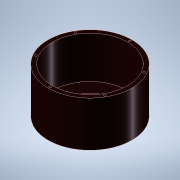
# Autodesk Inventor part: Top
Saved by Autodesk Inventor 2021 (Build 250183000, 183)
## iProperties
Created: 2022-09-01
Part Number: Top
Material: Ogólny
Document SubType Name: Modeling
Designer: MicnedSQ
Density: 1 g/cm^3
Appearance: Kasztanowa
Author: MicnedSQ
## iProperties of the stored document _Drukowanie 3D.ipt
Created: 2022-09-01
Part Number: _Drukowanie 3D
Material: Ogólny
Document SubType Name: Modeling
Designer: MicnedSQ
Density: 1 g/cm^3
Appearance: Domyślna
Author: MicnedSQ
Autodesk Inventor part; units mm, degrees
ref_plane "YZ Plane" through (0, 0, 0) normal (1, 0, 0) x (0, 1, 0)
ref_plane "XZ Plane" through (0, 0, 0) normal (0, 1, 0) x (-1, 0, 0)
ref_plane "XY Plane" through (0, 0, 0) normal (0, 0, 1) x (1, 0, 0)
sketch "Szkic1" plane through (0, 0, 0) normal (0, 1, 0) x (-1, 0, 0)
  circle A0 centre (0, 0) radius 75
  dimension "d0" = 150
  constraints: 1 centre point, 1 coincident
  measures "d0" diameter of A0
extrude "Wyciągnięcie proste1" add sketch "Szkic1" along normal blind 6
sketch "Szkic2" plane through (0, 6, 0) normal (0, 1, 0) x (1, 0, 0)
  circle A0 centre (0, 0) radius 26
  dimension "d3" = 52
  constraints: 1 centre point, 1 coincident
  measures "d3" diameter of A0
extrude "Wyciągnięcie proste2" cut sketch "Szkic2" against normal through all
sketch "Szkic4" plane through (0, 0, 0) normal (0, -1, 0) x (1, 0, 0)
  circle A0 centre (0, 0) radius 45
  circle A1 centre (0, 45) radius 3
  dimension "d10" = 90
  dimension "d11" = 6
  constraints: 1 centre point, 1 coincident, 1 vertical alignment, 2 other
  measures "d11" diameter of A1
extrude "Wyciągnięcie proste4" cut sketch "Szkic4" against normal blind 4 contours A1 A0 | A0 A1 picked at (-0.118, 43.9996) picked at (0.1052, 45.987)
sketch "Szkic5" plane through (0, 4, 45) normal (0, -1, 0) x (1, 0, 0)
  circle A0 centre (0, 0) radius 1.6
  point P0 (0, -45)
  dimension "d14" = 3.2
  constraints: 1 centre point
  measures "d14" diameter of A0
extrude "Wyciągnięcie proste5" cut sketch "Szkic5" against normal through all
pattern_circular "Szyk kołowy1" count 4 over 360 about axis through (0, 0, 0) along (0, 1, 0) of "Wyciągnięcie proste4", "Wyciągnięcie proste5"
sketch "Szkic6" plane through (0, 6, 0) normal (0, 1, 0) x (1, 0, 0)
  circle A0 centre (0, 0) radius 26
  circle A1 centre (0, 0) radius 32.5
  dimension "d20" = 65
  constraints: 2 centre point, 2 coincident
  measures "d20" diameter of A1
extrude "Wyciągnięcie proste6" cut sketch "Szkic6" against normal blind 4
sketch "Szkic7" plane through (0, 6, 0) normal (0, 1, 0) x (1, 0, 0)
  circle A0 centre (0, 0) radius 37.5
  circle A1 centre (0, 0) radius 32.5
  dimension "d23" = 75
  constraints: 2 centre point, 2 coincident
  measures "d23" diameter of A0
extrude "Wyciągnięcie proste7" add sketch "Szkic7" along normal blind 3
sketch "Szkic8" plane through (0, 6, 0) normal (0, 1, 0) x (1, 0, 0)
  circle A0 centre (0, 0) radius 75
  circle A1 centre (0, 0) radius 67.5
  dimension "d26" = 135
  dimension "d29" = 150
  constraints: 2 centre point, 2 coincident
  measures "d26" diameter of A1
  measures "d29" diameter of A0
extrude "Wyciągnięcie proste8" add sketch "Szkic8" along normal blind 75
sketch "Szkic9" plane through (0, 81, 0) normal (0, 1, 0) x (1, 0, 0)
  circle A0 centre (0, 0) radius 67.5 projected
  circle A1 centre (0, 0) radius 71.25
  circle A2 centre (0, 71.25) radius 1.95
  dimension "d30" = 142.5
  dimension "d31" = 3.9
  constraints: 1 centre point, 1 coincident, 1 vertical alignment, 2 other
  measures "d31" diameter of A2
extrude "Wyciągnięcie proste9" cut sketch "Szkic9" against normal blind 8 contours A2 A1 | A1 A2 picked at (0.0777, 70.6027) picked at (0.0743, 71.8938)
pattern_circular "Szyk kołowy2" count 6 over 360 about axis through (0, 0, 0) along (0, 1, 0) of "Wyciągnięcie proste9"
